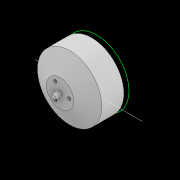
# Autodesk Inventor part: 3phaseMotor
Saved by Autodesk Inventor 2022.2 (Build 262287010, 287A)
## iProperties
Created: 2022-06-22
Part Number: 3phaseMotor
Material: Generic
Document SubType Name: Modeling
Designer: Árni Þór Þorgeirsson
Density: 1 g/cm^3
Appearance: Default
Author: Árni Þór Þorgeirsson
Autodesk Inventor part; units mm, degrees
ref_plane "YZ Plane" through (0, 0, 0) normal (1, 0, 0) x (0, 1, 0)
ref_plane "XZ Plane" through (0, 0, 0) normal (0, 1, 0) x (-1, 0, 0)
ref_plane "XY Plane" through (0, 0, 0) normal (0, 0, 1) x (1, 0, 0)
sketch "Sketch1" plane through (0, 0, 0) normal (0, 0, 1) x (1, 0, 0)
  circle A0 centre (0, 0) radius 29.5
  circle A1 centre (0, 0) radius 16 construction
  circle A2 centre (0, 0) radius 12.5 construction
  circle A3 centre (0, 0) radius 8.5
  line L0 (0, 0) -> (17.0589, 17.0589) construction
  line L1 (-45.7937, 0) -> (68.262, 0) projected
  line L2 (0, 0) -> (-17.0589, 17.0589) construction
  line L3 (0, 0) -> (-17.0589, -17.0589) construction
  line L4 (0, 0) -> (17.0589, -17.0589) construction
  line L5 (0, 0) -> (51.9684, 0) construction
  line L6 (0, 0) -> (-25.9842, 45.0059) construction
  line L7 (0, 0) -> (-25.9842, -45.0059) construction
  circle A4 centre (0, 0) radius 3 construction
  circle A5 centre (0, 0) radius 2 construction
  point P0 (8.5, 0)
  point P1 (-4.25, 7.3612)
  point P2 (-4.25, -7.3612)
  point P3 (8.8388, 8.8388)
  point P4 (-8.8388, -8.8388)
  point P5 (-8.8388, 8.8388)
  point P6 (8.8388, -8.8388)
  point P7 (16, 0)
  point P8 (-8, -13.8564)
  point P9 (-8, 13.8564)
  dimension "d0" = 59
  dimension "d1" = 32
  dimension "d2" = 25
  dimension "d3" = 17
  dimension "d4" = 45
  dimension "d8" = 360
  dimension "d12" = 360
  dimension "d14" = 6
  dimension "d15" = 4
  constraints: 14 end point, 11 point on line, 10 point on circle, 8 coincident, 6 centre point, 23 other
  measures "d0" diameter of A0
  measures "d1" diameter of A1
  measures "d2" diameter of A2
  measures "d3" diameter of A3
  measures "d4" angle of L1 L0
  measures "d14" diameter of A4
  measures "d15" diameter of A5
sketch "Sketch2" plane through (0, 0, 0) normal (0, 0, 1) x (1, 0, 0)
  circle A0 centre (0, 0) radius 29.5 projected
extrude "Extrusion1" add sketch "Sketch2" along normal mid plane 42.5
sketch "Sketch3" plane through (0, 0, 21.25) normal (0, 0, 1) x (1, 0, 0)
  circle A0 centre (0, 0) radius 2 projected
  circle A1 centre (0, 0) radius 29.5 projected
extrude "Extrusion2" cut sketch "Sketch3" against normal blind 6
sketch "Sketch4" plane through (0, 0, -21.25) normal (0, 0, -1) x (-1, 0, 0)
  circle A0 centre (0, 0) radius 3 projected
  circle A1 centre (0, 0) radius 29.5 projected
extrude "Extrusion3" cut sketch "Sketch4" against normal blind 3
sketch "Sketch5" plane through (0, 0, 15.25) normal (0, 0, 1) x (1, 0, 0)
  circle A0 centre (0, 0) radius 8.5 projected
  circle A1 centre (0, 0) radius 12.5
  point P0 (-4.25, 7.3612)
  point P1 (8.5, 0)
  point P2 (-4.25, -7.3612)
  dimension "d29" = 25
  constraints: 1 centre point, 1 coincident
  measures "d29" diameter of A1
hole "Hole1" at (-4.25, 7.3612, 15.25) at (8.5, 0, 15.25) at (-4.25, -7.3612, 15.25) direction (0, 0, -1) diameter 3 depth 5 tip angle 118
chamfer "Chamfer1" distance 8.8 distance2 17 1 edges at (-29.5, 0, 15.25) measured on face at (29.4043, -2.3738, -7.0833)
sketch "Sketch6" plane through (0, 0, -21.25) normal (0, 0, -1) x (-1, 0, 0)
  circle A0 centre (0, 0) radius 3 projected
extrude "Magnet" add sketch "Sketch6" along normal blind 2
chamfer "Chamfer2" distance 4.5 distance2 7.5 1 edges at (-29.5, 0, -18.25) measured on face at (29.118, -4.7321, -10.0167)
sketch "Sketch7" plane through (0, 0, -18.25) normal (0, 0, -1) x (-1, 0, 0)
  circle A0 centre (0, 0) radius 8.5 projected
  circle A1 centre (0, 0) radius 12.5 projected
  point P0 (8.8388, 8.8388)
  point P1 (-8.8388, 8.8388)
  point P2 (-8.8388, -8.8388)
  point P3 (8.8388, -8.8388)
  point P4 (8, 13.8564)
  point P5 (8, -13.8564)
  point P6 (-16, 0)
hole "Hole2" at (8.8388, 8.8388, -18.25) at (-8.8388, 8.8388, -18.25) at (-8.8388, -8.8388, -18.25) at (8.8388, -8.8388, -18.25) direction (0, 0, 1) diameter 3 depth 4 tip angle 118
hole "Hole3" at (-8, 13.8564, -18.25) at (16, 0, -18.25) at (-8, -13.8564, -18.25) direction (0, 0, 1) diameter 2.5 depth 3 tip angle 118
sketch "Sketch8" plane through (0, 0, -23.25) normal (0, 0, -1) x (-1, 0, 0)
  line L0 (-1.6203, 1.7761) -> (1.6105, 1.7761) construction
  line L1 (1.6105, 1.7761) -> (1.6105, -1.2719) construction
  line L2 (1.6105, -1.2719) -> (-1.6203, -1.2719) construction
  line L3 (-1.6203, -1.2719) -> (-1.6203, 1.7761) construction
  line L4 (1.3017, -1.2719) -> (0.8967, -1.2719)
  line L5 (0.8967, -1.2719) -> (0.8967, 1.3537)
  line L6 (0.8967, 1.3537) -> (0.1013, -0.4321)
  line L7 (0.1013, -0.4321) -> (-0.1457, -0.4321)
  line L8 (-0.1457, -0.4321) -> (-0.9336, 1.3537)
  line L9 (-0.9336, 1.3537) -> (-0.9336, -1.2719)
  line L10 (-0.9336, -1.2719) -> (-1.3115, -1.2719)
  line L11 (-1.3115, -1.2719) -> (-1.3115, 1.7761)
  line L12 (-1.3115, 1.7761) -> (-0.7583, 1.7761)
  line L13 (-0.7583, 1.7761) -> (0.0025, 0.0792)
  line L14 (0.0025, 0.0792) -> (0.7386, 1.7761)
  line L15 (0.7386, 1.7761) -> (1.3017, 1.7761)
  line L16 (1.3017, 1.7761) -> (1.3017, -1.2719)
  point P0 (0, 0)
  constraints: 2 other
extrude "Extrusion5" cut sketch "Sketch8" against normal blind 0.5
sketch "Sketch9" plane through (0, 0, -18.25) normal (0, 0, -1) x (-1, 0, 0)
  circle A0 centre (-8.8388, 8.8388) radius 1.5 projected
  circle A1 centre (8.8388, 8.8388) radius 1.5 projected
  circle A2 centre (8.8388, -8.8388) radius 1.5 projected
  circle A3 centre (-8.8388, -8.8388) radius 1.5 projected
  circle A4 centre (0, 0) radius 3 projected
  circle A5 centre (0, 0) radius 29.5 projected
  circle A6 centre (-16, 0) radius 1.25 projected
  circle A7 centre (8, 13.8564) radius 1.25 projected
  circle A8 centre (8, -13.8564) radius 1.25 projected
equation "\"d22\" = M3"
equation "\"d27\" = D5_M3"
equation "\"d38\" = M3"
equation "\"M3\" = 3"
equation "\"D5_M3\" = 5"
body "Solid1"
